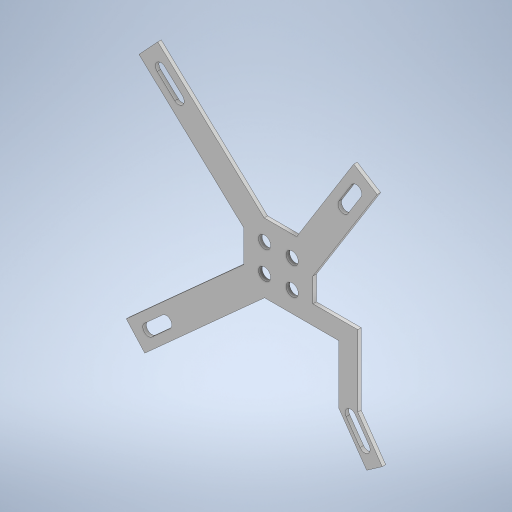
# Autodesk Inventor part: watercooler_fixed2
Saved by Autodesk Inventor 2023 (Build 270158000, 158)
## iProperties
Created: 2023-06-13
Part Number: watercooler_fixed2
Material: 一般
Document SubType Name: Sheet Metal
Designer: 310611102
Density: 1 g/cm^3
Sheet Metal Rule: Default_mm
Appearance: 預設
Author: 310611102
Autodesk Inventor part; units mm, degrees
ref_plane "YZ Plane" through (0, 0, 0) normal (1, 0, 0) x (0, 1, 0)
ref_plane "XZ Plane" through (0, 0, 0) normal (0, 1, 0) x (-1, 0, 0)
ref_plane "XY Plane" through (0, 0, 0) normal (0, 0, 1) x (1, 0, 0)
sketch "Sketch1" plane through (0, 0, 0) normal (0, 0, 1) x (1, 0, 0)
  line L0 (-10, 10) -> (10, 10)
  line L1 (10, 10) -> (10, -10)
  line L2 (10, -10) -> (-10, -10)
  line L3 (-10, -10) -> (-10, 10)
  line L4 (-10, 10) -> (10, -10) construction
  line L5 (10, 10) -> (-10, -10) construction
  circle A0 centre (-4, 4) radius 1.75
  line L6 (-4, 4) -> (0.2191, 4)
  line L7 (0.2191, 4) -> (0.2191, 2.6146)
  circle A1 centre (4, 4) radius 1.75
  circle A2 centre (-4, -4) radius 1.75
  circle A3 centre (4, -4) radius 1.75
  point P0 (0, 0)
  dimension "d0" = 20
  dimension "d1" = 20
  dimension "d2" = 3.5
  dimension "d5" = 8
  dimension "d8" = 8
  dimension "d11" = 4
  dimension "d12" = 4
  measures "d0" distance of L0.start L0.end
  measures "d1" distance of L0.end L1.end
  measures "d2" diameter of A0
  measures "d5" distance of L6.start A1.centre
  measures "d8" distance of L6.start A2.centre
  measures "d11" horizontal distance of point (0, 0) L6.start
  measures "d12" horizontal distance of point (0, 0) L6.start
extrude "Plate1" add sketch "Sketch1" along normal blind 1
sketch "Sketch2" plane through (0, 0, 1) normal (0, 0, 1) x (1, 0, 0)
  line L0 (-10, -10) -> (-10, 10)
  line L1 (-10, 10) -> (-33.9394, 32.3238)
  line L2 (-10, -10) -> (-37.6112, -34.8612)
  line L3 (-10, 10) -> (10, 10)
  line L4 (10, 10) -> (17.9255, 22.6834)
  line L5 (10, -10) -> (-10, -10)
  line L6 (-40.4218, 32.8995) -> (-8.9736, 3.5735)
  line L7 (-8.9736, 3.5735) -> (-3.5176, 9.4244)
  line L8 (-3.5176, 9.4244) -> (-34.9658, 38.7503)
  line L9 (-34.9658, 38.7503) -> (-40.4218, 32.8995)
  line L10 (-40.4218, 32.8995) -> (-3.5176, 9.4244) construction
  line L11 (-8.9736, 3.5735) -> (-34.9658, 38.7503) construction
  line L12 (10, 10) -> (10, -10)
  line L13 (-44.0946, -35.3164) -> (-8.8696, -3.5996)
  line L14 (-8.8696, -3.5996) -> (-3.5165, -9.5448)
  line L15 (-3.5165, -9.5448) -> (-38.7416, -41.2616)
  line L16 (-38.7416, -41.2616) -> (-44.0946, -35.3164)
  line L17 (-44.0946, -35.3164) -> (-3.5165, -9.5448) construction
  line L18 (-8.8696, -3.5996) -> (-38.7416, -41.2616) construction
  line L19 (28.6116, 32.2365) -> (9.9585, 2.3852)
  line L20 (9.9585, 2.3852) -> (3.1741, 6.6246)
  line L21 (3.1741, 6.6246) -> (21.8273, 36.4759)
  line L22 (21.8273, 36.4759) -> (28.6116, 32.2365)
  line L23 (28.6116, 32.2365) -> (3.1741, 6.6246) construction
  line L24 (9.9585, 2.3852) -> (21.8273, 36.4759) construction
  line L25 (23, -4.5) -> (10, -4.5)
  line L26 (10, -4.5) -> (10, -10)
  line L27 (10, -10) -> (23, -10)
  line L28 (23, -10) -> (23, -4.5)
  line L29 (23, -4.5) -> (10, -10) construction
  line L30 (10, -4.5) -> (23, -10) construction
  line L31 (17.5, -26.9397) -> (17.5, -10)
  line L32 (17.5, -10) -> (23, -10)
  line L33 (23, -10) -> (23, -30)
  line L34 (23, -30) -> (19.6429, -30)
  line L35 (16.1337, -34.9685) -> (23, -10) construction
  line L36 (17.5, -10) -> (23, -30) construction
  line L37 (25.5844, -38.4854) -> (17.5, -26.9397)
  line L38 (17.5, -26.9397) -> (22.0053, -23.785)
  line L39 (22.0053, -23.785) -> (30.0897, -35.3307)
  line L40 (30.0897, -35.3307) -> (25.5844, -38.4854)
  line L41 (25.5844, -38.4854) -> (22.0053, -23.785) construction
  line L42 (17.5, -26.9397) -> (30.0897, -35.3307) construction
  line L43 (23, -30) -> (23.7949, -31.1352)
  point P0 (0, 0)
  point P1 (-21.9697, 21.1619)
  point P2 (-23.8056, -22.4306)
  point P3 (15.8929, 19.4306)
  point P4 (16.5, -7.25)
  point P5 (20.25, -20)
  dimension "d14" = 137
  dimension "d15" = 138
  dimension "d17" = 148
  dimension "d18" = 8
  dimension "d19" = 8
  dimension "d21" = 8
  dimension "d22" = 42.5
  dimension "d23" = 7.3
  dimension "d24" = 9
  dimension "d25" = 9
  dimension "d28" = 56.4
  dimension "d29" = 52
  dimension "d35" = 5.5
  dimension "d36" = 5.5
  dimension "d38" = 13
  dimension "d39" = 20
  dimension "d41" = 5.5
  dimension "d42" = 145
  dimension "d43" = 46.2
  measures "d14" angle of L3 L1
  measures "d15" angle of L5 L2
  measures "d17" angle of L12 L4
  measures "d18" distance of L8.end L6.start
  measures "d19" distance of L21.end L19.start
  measures "d21" distance of L15.end L13.start
  measures "d22" distance from line of L22 point (0, 0)
  measures "d23" distance from line of L20 point (0, 0)
  measures "d24" distance from line of point (0, 0) L7
  measures "d25" distance from line of point (0, 0) L14
  measures "d28" distance from line of point (0, 0) L16
  measures "d29" distance from line of point (0, 0) L9
  measures "d35" distance of L5.start L25.end
  measures "d36" distance of L31.end L27.end
  measures "d38" distance of L25.start L25.end
  measures "d39" distance between parallel lines of L27 L34
  measures "d41" distance of L31.start L38.end
  measures "d42" angle of L33 L43
  measures "d43" distance from line of point (0, 0) L40
sheet face with bend "Face2" sketch "Sketch2" thickness 1 toward (0, 0, -1) bend radius 1 contours L5 L15 L16 L13 L0 | L0 L13 L14 L15 L5 | L6 L9 L8 L3 L0 | L0 L3 L8 L7 L6 | L12 L25 L28 L27 | L27 L33 L39 L38 L31 | L19 L20 L21 L3 L12 | L12 L3 L21 L22 L19 | L38 L39 L33 L34 L37 | L39 L40 L37 L34 L33
bend "Bend1"
sketch "Sketch4" plane through (0, 0, 1) normal (0, 0, 1) x (1, 0, 0)
  circle A0 centre (-32.5004, -30.2594) radius 1.6
  circle A1 centre (-37.7024, -34.9433) radius 1.6
  circle A2 centre (-34.037, 32.4149) radius 1.6
  circle A3 centre (-28.9175, 27.6409) radius 1.6
  circle A4 centre (22.5699, 30.116) radius 1.6
  circle A5 centre (18.8604, 24.1796) radius 1.6
  line L0 (-34.037, 32.4149) -> (-28.9175, 27.6409)
  line L1 (22.5699, 30.116) -> (18.8604, 24.1796)
  line L2 (-37.7024, -34.9433) -> (-32.5004, -30.2594)
  line L3 (20.9542, -27.0782) -> (24.9692, -32.8123)
  line L4 (30.0897, -35.3307) -> (23, -25.2055) projected
  circle A6 centre (20.9542, -27.0782) radius 1.6
  circle A7 centre (24.9692, -32.8123) radius 1.6
  line L5 (25.5844, -38.4854) -> (30.0897, -35.3307) projected
  line L6 (28.6116, 32.2365) -> (10, 2.4517) projected
  line L7 (-4.1349, 10) -> (-34.9658, 38.7503) projected
  line L8 (-44.0946, -35.3164) -> (-10, -4.6175) projected
  line L9 (-38.7416, -41.2616) -> (-44.0946, -35.3164) projected
  line L10 (21.8273, 36.4759) -> (28.6116, 32.2365) projected
  line L11 (-34.9658, 38.7503) -> (-40.4218, 32.8995) projected
  line L12 (-37.7024, -34.9433) -> (-32.5004, -30.2594) construction
  line L13 (-36.6318, -36.1324) -> (-31.4298, -31.4485)
  line L14 (-33.571, -29.0704) -> (-38.773, -33.7543)
  arc A8 (-38.773, -33.7543) -> (-36.6318, -36.1324) centre (-37.7024, -34.9433) ccw
  arc A9 (-31.4298, -31.4485) -> (-33.571, -29.0704) centre (-32.5004, -30.2594) ccw
  line L15 (20.9542, -27.0782) -> (24.9692, -32.8123) construction
  line L16 (19.6435, -27.996) -> (23.6585, -33.73)
  line L17 (26.2798, -31.8946) -> (22.2648, -26.1605)
  arc A10 (22.2648, -26.1605) -> (19.6435, -27.996) centre (20.9542, -27.0782) ccw
  arc A11 (23.6585, -33.73) -> (26.2798, -31.8946) centre (24.9692, -32.8123) ccw
  line L18 (18.8604, 24.1796) -> (22.5699, 30.116) construction
  line L19 (20.2173, 23.3318) -> (23.9267, 29.2681)
  line L20 (21.213, 30.9638) -> (17.5035, 25.0275)
  arc A12 (17.5035, 25.0275) -> (20.2173, 23.3318) centre (18.8604, 24.1796) ccw
  arc A13 (23.9267, 29.2681) -> (21.213, 30.9638) centre (22.5699, 30.116) ccw
  line L21 (-28.9175, 27.6409) -> (-34.037, 32.4149) construction
  line L22 (-27.8263, 28.8111) -> (-32.9458, 33.5851)
  line L23 (-35.1282, 31.2447) -> (-30.0087, 26.4707)
  arc A14 (-30.0087, 26.4707) -> (-27.8263, 28.8111) centre (-28.9175, 27.6409) ccw
  arc A15 (-32.9458, 33.5851) -> (-35.1282, 31.2447) centre (-34.037, 32.4149) ccw
  point P0 (0, 0)
  point P1 (-35.1014, -32.6014)
  point P2 (22.9617, -29.9453)
  point P3 (20.7151, 27.1478)
  point P4 (-31.4773, 30.0279)
  dimension "d54" = 2.75
  dimension "d55" = 3.2
  dimension "d56" = 3.2
  dimension "d58" = 5
  dimension "d59" = 7
  dimension "d60" = 3.2
  dimension "d61" = 3.2
  dimension "d62" = 3.2
  dimension "d63" = 3.2
  dimension "d64" = 3.2
  dimension "d65" = 3.2
  dimension "d66" = 8
  dimension "d67" = 8
  dimension "d68" = 8
  dimension "d69" = 5
  dimension "d70" = 7
  dimension "d71" = 5
  dimension "d72" = 7
  dimension "d73" = 5
  dimension "d74" = 7
  constraints: 42 end point, 16 centre point, 16 point on circle, 16 tangent, 8 midpoint, 8 parallel, 6 coincident, 4 collinear, 4 concentric
  measures "d54" distance between parallel lines of L4 L3
  measures "d55" diameter of A6
  measures "d56" diameter of A7
  measures "d58" distance from line of L5 L3.end
  measures "d59" distance of L3.start L3.end
  measures "d60" diameter of A0
  measures "d61" diameter of A1
  measures "d62" diameter of A5
  measures "d63" diameter of A4
  measures "d64" diameter of A3
  measures "d65" diameter of A2
  measures "d66" diameter of L6 L1
  measures "d67" diameter of L7 L0
  measures "d68" diameter of L8 L2
  measures "d69" distance from line of L9 A1.centre
  measures "d70" distance of L2.start L2.end
  measures "d71" distance from line of L10 A4.centre
  measures "d72" distance of L1.start L1.end
  measures "d73" distance from line of L11 A2.centre
  measures "d74" distance of L0.start L0.end
extrude "Cut1" cut sketch "Sketch4" against normal blind 1
sketch "Sketch3" plane through (-41.7142, -43.9381, 0) normal (-0.7431448, -0.6691306, 0) x (0.6691306, -0.7431448, 0)
  line L0 (-8, 0) -> (0, 0)
  line L1 (0, 0) -> (0, 25)
  line L2 (0, 25) -> (-8, 25)
  line L3 (-8, 25) -> (-8, 0)
  constraints: 6 end point, 1 horizontal, 1 perpendicular, 1 vertical
equation "\"d75\" = 厚度"
equation "\"d13\" = 厚度"
equation "\"d30\" = 折彎半徑"
equation "\"d31\" = 折彎離隙寬度"
equation "\"d33\" = 最小剩餘"
equation "\"d32\" = 折彎離隙深度"
equation "\"d34\" = 轉移半徑"
equation "\"折彎半徑\" = 厚度"
equation "\"折彎離隙寬度\" = 厚度"
equation "\"折彎離隙深度\" = 0.5 * 厚度"
equation "\"轉角離隙大小\" = 4 * 厚度"
equation "\"最小剩餘\" = 2 * 厚度"
equation "\"轉移半徑\" = 折彎半徑"
equation "\"Jacobi半徑大小\" = 折彎半徑"
equation "\"間隙大小\" = 厚度"
equation "\"厚度\" = 1"
body "Solid1"
